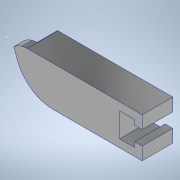
# Autodesk Inventor part: Finray_test_8_Kerbe_20deg_V4_links
Saved by Autodesk Inventor 2022 (Build 260153000, 153)
## iProperties
Created: 2022-02-28
Part Number: Finray_test_8_Kerbe_20deg_V4_links
Material: Generic
Document SubType Name: Modeling
Designer: richa
Density: 1 g/cm^3
Appearance: Aluminum - Flat
Author: richa
Autodesk Inventor part; units mm, degrees
ref_plane "YZ Plane" through (0, 0, 0) normal (1, 0, 0) x (0, 1, 0)
ref_plane "XZ Plane" through (0, 0, 0) normal (0, 1, 0) x (-1, 0, 0)
ref_plane "XY Plane" through (0, 0, 0) normal (0, 0, 1) x (1, 0, 0)
sketch "Sketch5" plane through (0, 0, 0) normal (0, 0, 1) x (1, 0, 0)
  line L0 (52.8, -15.6) -> (52.8, -10.6)
  line L1 (52.8, -10.6) -> (49.8, -10.6)
  line L2 (49.8, -10.6) -> (49.8, -12.55)
  line L3 (44, -12.55) -> (44, -3.05)
  line L4 (49.8, -3.05) -> (49.8, -5)
  line L5 (49.8, -5) -> (52.8, -5)
  line L6 (52.8, -5) -> (52.8, 0)
  line L7 (52.8, 0) -> (7.8, 0)
  line L8 (44, -3.05) -> (49.8, -3.05)
  line L9 (44, -12.55) -> (49.8, -12.55)
  line L10 (52.8, -15.6) -> (7.8, -15.6)
  arc A0 (7.8, 0) -> (7.8, -15.6) centre (7.8, -7.8) ccw
  point P0 (0, 0)
  dimension "d41" = 5.8
  dimension "d48" = 44
  dimension "d63" = 45
  dimension "d67" = 15.6
  dimension "d71" = 0
  dimension "d72" = 36.2
  dimension "d85" = 5.6
  dimension "d86" = 9.5
  dimension "d87" = 3
  constraints: 22 end point, 7 perpendicular, 4 collinear, 2 parallel, 2 point on circle, 2 tangent, 1 centre point, 1 horizontal, 1 vertical
  measures "d41" distance between parallel lines of L2 L3
  measures "d48" distance from line of L3 point (0, 0)
  measures "d63" distance of L0.start L10.end
  measures "d67" diameter of A0
  measures "d71" distance from line of point (0, 0) L7
  measures "d72" distance from line of L3 A0.centre
  measures "d85" distance between parallel lines of L1 L5
  measures "d86" distance of L3.start L3.end
  measures "d87" distance of L4.end L5.end
extrude "Extrusion2" add sketch "Sketch5" along normal blind 12
sketch "Sketch9" plane through (0, 0, 12) normal (0, 0, 1) x (1, 0, 0)
  line L0 (52.8, 0) -> (7.8, 0) projected
  line L1 (7.6933, 0) -> (9.4034, -4.6985)
  line L2 (9.4034, -4.6985) -> (0.0065, -8.1187)
  arc A0 (7.8, 0) -> (7.8, -15.6) centre (7.8, -7.8) ccw projected
  point P0 (0, 0)
  point P1 (7.6936, -0.0007)
  dimension "d89" = 5
  dimension "d92" = 110
  dimension "d93" = 10
  constraints: 4 end point, 1 perpendicular, 1 point on circle, 1 point on line
  measures "d89" distance of L1.start L1.end
  measures "d92" angle of L0 L1
  measures "d93" distance of L1.end L2.end
extrude "Extrusion6" cut sketch "Sketch9" along normal blind 8 from surface at -12
sketch "Sketch11" plane through (0, 0, 12) normal (0, 0, 1) x (1, 0, 0)
  line L0 (1.7497, 0.249) -> (7.6768, -16.0354)
  line L1 (7.6768, -16.0354) -> (-2.2601, -19.6521)
  line L2 (-2.2601, -19.6521) -> (-8.1871, -3.3677)
  line L3 (-8.1871, -3.3677) -> (1.7497, 0.249)
  line L4 (7.6936, -0.0007) -> (9.4034, -4.6985) projected
  point P0 (0, 0)
  dimension "d98" = 5.5
  constraints: 8 end point, 3 perpendicular, 1 parallel
  measures "d98" distance between parallel lines of L0 L4
extrude "Extrusion8" cut sketch "Sketch11" against normal through all
fillet "Fillet2" radius 15 1 edges at (7.5164, -15.5948, 6)
sketch "Sketch12" plane through (0, 0, 12) normal (0, 0, 1) x (1, 0, 0)
  point P0 (0, 0)
equation "\"l1\" = 8"
body "Solid2"
